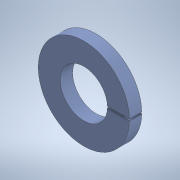
# Autodesk Inventor part: Arandela Grower m6
Saved by Autodesk Inventor 2020 (Build 240168000, 168)
## iProperties
Created: 2020-05-19
Part Number: Arandela Grower m6
Material: Generic
Document SubType Name: Modeling
Designer: Dante
Density: 1 g/cm^3
Appearance: Default
Mass: 0.127303 g
Surface Area: 2.57586 cm^2
Volume: 0.127303 cm^3
Author: Dante
Autodesk Inventor part; units mm, degrees
ref_plane "YZ Plane" through (0, 0, 0) normal (1, 0, 0) x (0, 1, 0)
ref_plane "XZ Plane" through (0, 0, 0) normal (0, 1, 0) x (-1, 0, 0)
ref_plane "XY Plane" through (0, 0, 0) normal (0, 0, 1) x (1, 0, 0)
sketch "Sketch1" plane through (0, 0, 0) normal (0, 0, 1) x (1, 0, 0)
  circle A0 centre (0, 0) radius 3.05
  circle A1 centre (0, 0) radius 5.9
  dimension "d0" = 6.1
  dimension "d1" = 11.8
  constraints: 2 centre point, 2 coincident
  measures "d0" diameter of A0
  measures "d1" diameter of A1
extrude "Extrusion1" add sketch "Sketch1" along normal blind 1.6
sketch "Sketch2" plane through (0, 0, 0) normal (0, 0, -1) x (-1, 0, 0)
  circle A0 centre (0, 0) radius 3.05 projected
  line L0 (-3.05, 0.1) -> (-5.9, 0.1)
  circle A1 centre (0, 0) radius 5.9 projected
  line L1 (-5.9, 0) -> (-5.9, 0.1)
  line L2 (-3.05, 0.1) -> (-3.0398, 0.1)
  line L3 (-3.0398, 0.1) -> (-3.0398, -0.8229)
  line L4 (-3.0398, 0) -> (-3.0138, 0)
  line L5 (-3.05, -0.1) -> (-5.9, -0.1)
  line L6 (-5.9, 0) -> (-5.9, -0.1)
  line L7 (-3.05, -0.1) -> (-3.0398, -0.1)
  line L8 (-3.0398, -0.1) -> (-3.0398, 0.8229)
  point P0 (-5.8992, -0.1)
  point P1 (-3.0484, -0.1)
  point P2 (-3.0484, 0.1)
  point P3 (-5.8992, 0.1)
  constraints: 18 end point, 4 symmetric about line, 3 horizontal, 1 perpendicular, 1 point on line, 1 vertical, 2 other
extrude "Extrusion2" cut sketch "Sketch2" against normal blind 10 contours A0 L5 A1 L0 picked at (-3.9998, -0.0667)
body "Solid1"
